Autodesk Inventor part; units mm, degrees
(part 2 of 2)
  line L1117 (7.1, 50) -> (57.9, 50)
  line L1118 (57.9, 50) -> (57.9, 55)
  line L1119 (57.9, 55) -> (7.1, 55)
  line L1120 (7.1, 55) -> (7.1, 50)
  line L1121 (88, 20.43) -> (70.5, 20.43)
  line L1122 (70.5, 20.43) -> (70.5, 33.57)
  line L1123 (70.5, 33.57) -> (88, 33.57)
  line L1124 (88, 33.57) -> (88, 34.25)
  line L1125 (88, 34.25) -> (87.7, 34.25)
  line L1126 (87.7, 34.25) -> (87.7, 33.57)
  line L1127 (88, 20.43) -> (88, 19.75)
  line L1128 (88, 19.75) -> (87.7, 19.75)
  line L1129 (87.7, 19.75) -> (87.7, 20.43)
  line L1130 (32.275, 6.675) -> (31.125, 6.675)
  line L1131 (31.125, 6.675) -> (31.125, 5.525)
  line L1132 (31.125, 5.525) -> (32.275, 5.525)
  line L1133 (32.275, 5.525) -> (32.275, 6.675)
  arc A46 (32.2, 5.7) -> (32, 5.7) centre (32.1, 5.7) ccw
  arc A47 (32, 5.7) -> (32.2, 5.7) centre (32.1, 5.7) ccw
  line L1134 (55.5, 35) -> (55.5, 41)
  point P0 (0, 0)
  point P1 (5, 80)
  constraints: 2270 end point, 592 point on line, 80 point on circle, 48 centre point, 4 midpoint, 1 other
extrude "押し出し1" add sketch "スケッチ1" along normal blind 1.6 contours A0 | A2 L149 L150 L161 L160 | L160 L161 L150 A2 | A2 L150 L159 L160 | L149 L152 L151 L150 A2 | A2 L150 L149 | L153 L154 L155 L149 | L156 L157 L158 L152 | A4 | A6 | L135 L134 L133 L0 | L0 L20 L19 L18 L29 L28 L27 L78 L79 L80 A11 L3 A10 L2 A9 L107 L108 L109 L1 L1123 L1122 L1121 L197 L196 L195 A8 L133 L134 L135 | L0 L18 L19 L20 | L0 L27 L28 L29 | L195 L196 L197 L1 A8 | L0 L80 L79 L78 | L1121 L1122 L1123 L1 | L109 L108 L107 A9 L1 | L7 L6 L5 L4 | A13 A12 | L11 L17 L15 L12 L13 L14 L16 L10 L9 L8 | L11 L16 L15 L17 | L15 L14 L13 L12 | L39 L38 L37 L36 | L43 L42 L41 L40 | L47 L48 L45 L44 | L47 L49 L45 L48 | L47 L46 L45 L49 | L53 L52 L51 L50 | A15 A14 | L57 L56 L55 L54 | A17 A16 | L60 L59 L58 | L59 L63 L62 L61 L64 | L68 L69 L66 L65 | L68 L70 L66 L69 | L68 L67 L66 L70 | L74 L75 L72 L71 | L74 L76 L72 L75 | L74 L73 L72 L76 | L81 L82 L83 L84 L85 L86 L87 L88 | L92 L93 L102 L89 | L102 L93 L94 L95 L91 L104 L89 | L92 L95 L102 L93 | L104 L91 L90 L98 L97 L96 L89 | L102 L95 L94 L93 | L92 L91 L102 L95 | L96 L97 L98 L90 | L117 L118 L119 L120 L116 L115 L114 L113 L112 L111 L110 | L117 L120 L119 L118 | L128 L129 L130 L131 L127 L126 L125 L124 L123 L122 L121 | L128 L131 L130 L129 | L143 L142 L141 L140 | L145 L146 L147 L148 | A19 A18 | A21 A20 | A23 A22 | L166 L165 L164 L162 | L162 L164 L163 L166 | L163 L164 L167 L166 | A25 A24 | L172 L171 L170 L168 | L168 L170 L169 L172 | L169 L170 L173 L172 | A27 A26 | L178 L177 L176 L174 | L174 L176 L175 L178 | L175 L176 L179 L178 | A29 A28 | L184 L183 L182 L180 | L180 L182 L181 L184 | L181 L182 L185 L184 | A31 A30 | L189 L188 L187 L186 | A33 A32 | L190 L191 L192 L193 L194 | L204 L205 L206 L207 | L211 L212 L209 L208 | L211 L213 L209 L212 | L211 L210 L209 L213 | L217 L218 L215 L214 | L217 L219 L215 L218 | L217 L216 L215 L219 | L223 L224 L221 L220 | L223 L225 L221 L224 | L223 L222 L221 L225 | L229 L230 L227 L226 | L229 L231 L227 L230 | L229 L228 L227 L231 | L235 L236 L233 L232 | L235 L237 L233 L236 | L235 L234 L233 L237 | L241 L242 L239 L238 | L241 L243 L239 L242 | L241 L240 L239 L243 | L247 L248 L245 L244 | L247 L249 L245 L248 | L247 L246 L245 L249 | L253 L254 L251 L250 | L253 L255 L251 L254 | L253 L252 L251 L255 | L259 L260 L257 L256 | L259 L261 L257 L260 | L259 L258 L257 L261 | L265 L266 L263 L262 | L265 L267 L263 L266 | L265 L264 L263 L267 | L271 L272 L269 L268 | L271 L273 L269 L272 | L271 L270 L269 L273 | L277 L278 L275 L274 | L277 L279 L275 L278 | L277 L276 L275 L279 | L283 L284 L281 L280 | L283 L285 L281 L284 | L283 L282 L281 L285 | L289 L290 L287 L286 | L289 L291 L287 L290 | L289 L288 L287 L291 | L295 L296 L293 L292 | L295 L297 L293 L296 | L295 L294 L293 L297 | L301 L302 L299 L298 | L301 L303 L299 L302 | L301 L300 L299 L303 | L307 L308 L305 L304 | L307 L309 L305 L308 | L307 L306 L305 L309 | L313 L314 L311 L310 | L313 L315 L311 L314 | L313 L312 L311 L315 | L319 L320 L317 L316 | L319 L321 L317 L320 | L319 L318 L317 L321 | L325 L326 L323 L322 | L325 L327 L323 L326 | L325 L324 L323 L327 | L331 L332 L329 L328 | L331 L333 L329 L332 | L331 L330 L329 L333 | L337 L338 L335 L334 | L337 L339 L335 L338 | L337 L336 L335 L339 | L343 L344 L341 L340 | L343 L345 L341 L344 | L343 L342 L341 L345 | L346 L350 L348 L349 | L346 L351 L348 L350 | L346 L347 L348 L351 | L352 L356 L354 L355 | L352 L357 L354 L356 | L352 L353 L354 L357 | L358 L362 L360 L361 | L358 L363 L360 L362 | L358 L359 L360 L363 | L364 L368 L366 L367 | L364 L369 L366 L368 | L364 L365 L366 L369 | L370 L374 L372 L373 | L370 L375 L372 L374 | L370 L371 L372 L375 | L376 L380 L378 L379 | L376 L381 L378 L380 | L376 L377 L378 L381 | L382 L386 L384 L385 | L382 L387 L384 L386 | L382 L383 L384 L387 | L388 L392 L390 L391 | L388 L393 L390 L392 | L388 L389 L390 L393 | L394 L398 L396 L397 | L394 L399 L396 L398 | L394 L395 L396 L399 | L403 L404 L401 L400 | L403 L405 L401 L404 | L403 L402 L401 L405 | L409 L410 L407 L406 | L409 L411 L407 L410 | L409 L408 L407 L411 | L415 L416 L413 L412 | L415 L417 L413 L416 | L415 L414 L413 L417 | L421 L422 L419 L418 | L421 L423 L419 L422 | L421 L420 L419 L423 | L427 L428 L425 L424 | L427 L429 L425 L428 | L427 L426 L425 L429 | L433 L434 L431 L430 | L433 L435 L431 L434 | L433 L432 L431 L435 | L439 L440 L437 L436 | L439 L441 L437 L440 | L439 L438 L437 L441 | L445 L446 L443 L442 | L445 L447 L443 L446 | L445 L444 L443 L447 | L452 L451 L450 L448 | L448 L450 L449 L452 | L449 L450 L453 L452 | L458 L457 L456 L454 | L454 L456 L455 L458 | L455 L456 L459 L458 | L464 L463 L462 L460 | L460 L462 L461 L464 | L461 L462 L465 L464 | L470 L469 L468 L466 | L466 L468 L467 L470 | L467 L468 L471 L470 | L476 L475 L474 L472 | L472 L474 L473 L476 | L473 L474 L477 L476 | L482 L481 L480 L478 | L478 L480 L479 L482 | L479 L480 L483 L482 | L488 L487 L486 L484 | L484 L486 L485 L488 | L485 L486 L489 L488 | L494 L493 L492 L490 | L490 L492 L491 L494 | L491 L492 L495 L494 | L500 L499 L498 L496 | L496 L498 L497 L500 | L497 L498 L501 L500 | L506 L505 L504 L502 | L502 L504 L503 L506 | L503 L504 L507 L506 | L512 L511 L510 L508 | L508 L510 L509 L512 | L509 L510 L513 L512 | L518 L517 L516 L514 | L514 L516 L515 L518 | L515 L516 L519 L518 | L524 L523 L522 L520 | L520 L522 L521 L524 | L521 L522 L525 L524 | L530 L529 L528 L526 | L526 L528 L527 L530 | L527 L528 L531 L530 | L536 L535 L534 L532 | L532 L534 L533 L536 | L533 L534 L537 L536 | L542 L541 L540 L538 | L538 L540 L539 L542 | L539 L540 L543 L542 | L548 L547 L546 L544 | L544 L546 L545 L548 | L545 L546 L549 L548 | L553 L552 L551 L550 | A35 A34 | L557 L556 L555 L554 | A37 A36 | L561 L560 L562 L558 | L562 L560 L563 L558 | L563 L560 L559 L558 | L567 L566 L568 L564 | L568 L566 L569 L564 | L569 L566 L565 L564 | L573 L572 L574 L570 | L574 L572 L575 L570 | L575 L572 L571 L570 | L579 L578 L580 L576 | L580 L578 L581 L576 | L581 L578 L577 L576 | L585 L584 L586 L582 | L586 L584 L587 L582 | L587 L584 L583 L582 | L591 L590 L592 L588 | L592 L590 L593 L588 | L593 L590 L589 L588 | L597 L596 L598 L594 | L598 L596 L599 L594 | L599 L596 L595 L594 | L603 L602 L604 L600 | L604 L602 L605 L600 | L605 L602 L601 L600 | L609 L608 L610 L606 | L610 L608 L611 L606 | L611 L608 L607 L606 | L615 L614 L616 L612 | L616 L614 L617 L612 | L617 L614 L613 L612 | L621 L620 L622 L618 | L622 L620 L623 L618 | L623 L620 L619 L618 | L627 L626 L628 L624 | L628 L626 L629 L624 | L629 L626 L625 L624 | L633 L632 L634 L630 | L634 L632 L635 L630 | L635 L632 L631 L630 | L639 L638 L640 L636 | L640 L638 L641 L636 | L641 L638 L637 L636 | L645 L644 L646 L642 | L646 L644 L647 L642 | L647 L644 L643 L642 | L651 L650 L652 L648 | L652 L650 L653 L648 | L653 L650 L649 L648 | L657 L656 L658 L654 | L658 L656 L659 L654 | L659 L656 L655 L654 | L663 L662 L664 L660 | L664 L662 L665 L660 | L665 L662 L661 L660 | L669 L668 L670 L666 | L670 L668 L671 L666 | L671 L668 L667 L666 | L675 L674 L676 L672 | L676 L674 L677 L672 | L677 L674 L673 L672 | L681 L680 L682 L678 | L682 L680 L683 L678 | L683 L680 L679 L678 | L687 L686 L688 L684 | L688 L686 L689 L684 | L689 L686 L685 L684 | L693 L692 L694 L690 | L694 L692 L695 L690 | L695 L692 L691 L690 | L699 L698 L700 L696 | L700 L698 L701 L696 | L701 L698 L697 L696 | L705 L704 L706 L702 | L706 L704 L707 L702 | L707 L704 L703 L702 | L711 L710 L712 L708 | L712 L710 L713 L708 | L713 L710 L709 L708 | L717 L716 L718 L714 | L718 L716 L719 L714 | L719 L716 L715 L714 | L723 L722 L724 L720 | L724 L722 L725 L720 | L725 L722 L721 L720 | L729 L728 L730 L726 | L730 L728 L731 L726 | L731 L728 L727 L726 | L735 L734 L736 L732 | L736 L734 L737 L732 | L737 L734 L733 L732 | L741 L740 L742 L738 | L742 L740 L743 L738 | L743 L740 L739 L738 | L747 L746 L748 L744 | L748 L746 L749 L744 | L749 L746 L745 L744 | L753 L752 L754 L750 | L754 L752 L755 L750 | L755 L752 L751 L750 | L759 L758 L760 L756 | L760 L758 L761 L756 | L761 L758 L757 L756 | L765 L764 L766 L762 | L766 L764 L767 L762 | L767 L764 L763 L762 | L771 L770 L772 L768 | L772 L770 L773 L768 | L773 L770 L769 L768 | L777 L776 L778 L774 | L778 L776 L779 L774 | L779 L776 L775 L774 | L783 L782 L784 L780 | L784 L782 L785 L780 | L785 L782 L781 L780 | L789 L788 L790 L786 | L790 L788 L791 L786 | L791 L788 L787 L786 | L795 L794 L796 L792 | L796 L794 L797 L792 | L797 L794 L793 L792 | L801 L800 L802 L798 | L802 L800 L803 L798 | L803 L800 L799 L798 | L807 L806 L808 L804 | L808 L806 L809 L804 | L809 L806 L805 L804 | L810 L814 L812 L813 | L810 L815 L812 L814 | L810 L811 L812 L815 | L816 L817 L818 L819 | L820 L821 L822 L823 | L823 L826 L825 L824 | L831 L832 L833 L821 | L823 L830 L829 L828 | L834 L844 L836 L837 | L850 L993 L848 L847 L846 L834 | L834 L845 L836 L844 | L834 L835 L836 L845 | L840 L839 L838 | L851 L861 L853 L854 | L867 L866 L865 L864 L863 L851 | L851 L862 L853 L861 | L851 L852 L853 L862 | L857 L856 L855 | L871 L872 L873 L874 L870 L880 L868 | L880 L870 L882 L868 | L872 L875 L874 L871 | L871 L874 L873 L872 | L882 L870 L869 L878 L877 L876 L868 | L876 L877 L878 L869 | L869 L878 L879 L876 | L884 L894 L886 L887 | L884 L896 L886 L894 | L887 L890 L889 L888 | L884 L885 L886 L896 | L891 L892 L893 L885 | L901 L900 L899 L898 | L898 L908 L907 L906 | L912 L913 L914 L900 | L898 L911 L910 L909 | L905 L904 L903 L902 | L918 L917 L916 L915 | L915 L925 L924 L923 | L929 L930 L931 L917 | L915 L928 L927 L926 | L922 L921 L920 L919 | L935 L934 L933 L932 | L932 L942 L941 L940 | L949 L950 L951 L934 | L932 L945 L944 L943 | L955 L956 L957 L934 | L932 L948 L947 L946 | L952 L953 L954 L934 | L939 L938 L937 L936 | A39 A38 | L961 L960 L959 L958 | L958 L968 L967 L966 | L976 L977 L975 L960 | L958 L971 L970 L969 | L978 L979 L983 L960 | L958 L974 L973 L972 | L980 L981 L982 L960 | L965 L964 L963 L962 | L988 L987 L986 L985 L984 | L992 L991 L990 L989 | A41 A40 | L994 L995 L996 L1134 | A43 A42 | L1000 L1001 L998 L997 | L1000 L1002 L998 L1001 | L1000 L999 L998 L1002 | L1006 L1007 L1004 L1003 | L1006 L1008 L1004 L1007 | L1006 L1005 L1004 L1008 | L1012 L1013 L1010 L1009 | L1012 L1014 L1010 L1013 | L1012 L1011 L1010 L1014 | L1018 L1019 L1016 L1015 | L1018 L1020 L1016 L1019 | L1018 L1017 L1016 L1020 | L1024 L1025 L1022 L1021 | L1024 L1026 L1022 L1025 | L1024 L1023 L1022 L1026 | L1030 L1031 L1028 L1027 | L1030 L1032 L1028 L1031 | L1030 L1029 L1028 L1032 | L1036 L1037 L1034 L1033 | L1036 L1038 L1034 L1037 | L1036 L1035 L1034 L1038 | L1042 L1043 L1040 L1039 | L1042 L1044 L1040 L1043 | L1042 L1041 L1040 L1044 | L1048 L1049 L1046 L1045 | L1048 L1050 L1046 L1049 | L1048 L1047 L1046 L1050 | L1054 L1055 L1052 L1051 | L1054 L1056 L1052 L1055 | L1054 L1053 L1052 L1056 | L1060 L1059 L1061 L1057 | L1061 L1059 L1062 L1057 | L1062 L1059 L1058 L1057 | L1066 L1065 L1067 L1063 | L1067 L1065 L1068 L1063 | L1068 L1065 L1064 L1063 | L1072 L1071 L1073 L1069 | L1073 L1071 L1074 L1069 | L1074 L1071 L1070 L1069 | L1078 L1077 L1079 L1075 | L1079 L1077 L1080 L1075 | L1080 L1077 L1076 L1075 | L1084 L1083 L1082 L1081 | L1081 L1091 L1090 L1089 | L1098 L1099 L1100 L1083 | L1081 L1094 L1093 L1092 | L1101 L1102 L1103 L1083 | L1081 L1097 L1096 L1095 | L1088 L1087 L1086 L1085 | L1104 L1105 L1106 L1107 | A45 A44 | L1112 L1111 L1110 L1109 L1108 | L1116 L1115 L1114 L1113 | L1120 L1119 L1118 L1117 | L1133 L1132 L1131 L1130 | A47 A46
extrude "押し出し2" add sketch "スケッチ1" against normal blind 5 contours L135 L134 L133 L0 | L0 L137 L136 L139
extrude "押し出し3" add sketch "スケッチ1" against normal blind 15 contours L195 L196 L197 L1 A8 | A8 L1 L197 L198 L195 | L1121 L1122 L1123 L1 | L1 L1123 L849 L1121
extrude "押し出し4" add sketch "スケッチ1" against normal blind 12 contours L109 L108 L107 A9 L1 | L1 A9 L107 L106 L109
extrude "押し出し5" add sketch "スケッチ1" against normal blind 2 contours L78 L77 L80 L0 | L0 L80 L79 L78 | L15 L14 L13 L12 | L39 L38 L37 L36 | L43 L42 L41 L40 | L59 L63 L62 L61 L64 | L166 L165 L164 L162 | L162 L164 L163 L166 | L163 L164 L167 L166 | A25 A24 | L172 L171 L170 L168 | L168 L170 L169 L172 | L169 L170 L173 L172 | A27 A26 | L178 L177 L176 L174 | L174 L176 L175 L178 | L175 L176 L179 L178 | A29 A28 | L184 L183 L182 L180 | L180 L182 L181 L184 | L181 L182 L185 L184 | A31 A30 | L189 L188 L187 L186 | A33 A32 | L190 L191 L192 L193 L194 | L403 L404 L401 L400 | L403 L405 L401 L404 | L403 L402 L401 L405 | L409 L410 L407 L406 | L409 L411 L407 L410 | L409 L408 L407 L411 | L415 L416 L413 L412 | L415 L417 L413 L416 | L415 L414 L413 L417 | L421 L422 L419 L418 | L421 L423 L419 L422 | L421 L420 L419 L423 | L427 L428 L425 L424 | L427 L429 L425 L428 | L427 L426 L425 L429 | L433 L434 L431 L430 | L433 L435 L431 L434 | L433 L432 L431 L435 | L439 L440 L437 L436 | L439 L441 L437 L440 | L439 L438 L437 L441 | L452 L451 L450 L448 | L448 L450 L449 L452 | L449 L450 L453 L452 | L458 L457 L456 L454 | L454 L456 L455 L458 | L455 L456 L459 L458 | L494 L493 L492 L490 | L490 L492 L491 L494 | L491 L492 L495 L494 | L500 L499 L498 L496 | L496 L498 L497 L500 | L497 L498 L501 L500 | L506 L505 L504 L502 | L502 L504 L503 L506 | L503 L504 L507 L506 | L512 L511 L510 L508 | L508 L510 L509 L512 | L509 L510 L513 L512 | L518 L517 L516 L514 | L514 L516 L515 L518 | L515 L516 L519 L518 | L524 L523 L522 L520 | L520 L522 L521 L524 | L521 L522 L525 L524 | L530 L529 L528 L526 | L526 L528 L527 L530 | L527 L528 L531 L530 | L536 L535 L534 L532 | L532 L534 L533 L536 | L533 L534 L537 L536 | L542 L541 L540 L538 | L538 L540 L539 L542 | L539 L540 L543 L542 | L548 L547 L546 L544 | L544 L546 L545 L548 | L545 L546 L549 L548 | L681 L680 L682 L678 | L682 L680 L683 L678 | L683 L680 L679 L678 | L687 L686 L688 L684 | L688 L686 L689 L684 | L689 L686 L685 L684 | L693 L692 L694 L690 | L694 L692 L695 L690 | L695 L692 L691 L690 | L699 L698 L700 L696 | L700 L698 L701 L696 | L701 L698 L697 L696 | L705 L704 L706 L702 | L706 L704 L707 L702 | L707 L704 L703 L702 | L711 L710 L712 L708 | L712 L710 L713 L708 | L713 L710 L709 L708 | L765 L764 L766 L762 | L766 L764 L767 L762 | L767 L764 L763 L762 | L771 L770 L772 L768 | L772 L770 L773 L768 | L773 L770 L769 L768 | L777 L776 L778 L774 | L778 L776 L779 L774 | L779 L776 L775 L774 | L783 L782 L784 L780 | L784 L782 L785 L780 | L785 L782 L781 L780 | L789 L788 L790 L786 | L790 L788 L791 L786 | L791 L788 L787 L786 | L795 L794 L796 L792 | L796 L794 L797 L792 | L797 L794 L793 L792 | L810 L814 L812 L813 | L810 L815 L812 L814 | L810 L811 L812 L815 | L988 L987 L986 L985 L984 | L992 L991 L990 L989 | L994 L995 L996 L1134 | L1112 L1111 L1110 L1109 L1108 | L1116 L1115 L1114 L1113
extrude "押し出し6" add sketch "スケッチ1" against normal blind 3 contours L20 L21 L18 L0 | L0 L18 L19 L20 | L26 L25 L24 L23 L22 L21 | L29 L30 L27 L0 | L0 L27 L28 L29 | L35 L34 L33 L32 L31 L30
extrude "押し出し7" add sketch "スケッチ1" against normal blind 10 contours L1120 L1119 L1118 L1117
